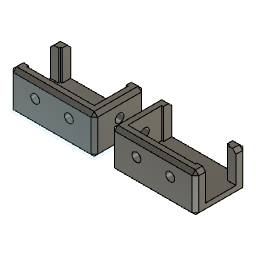
Footv2.5 (Autodesk Fusion 360 design; units mm, degrees)
part number: FootR
part number: FootL
Autodesk Fusion 360 part; units mm, degrees
sketch "Sketch1" plane through (0, 0, 0) normal (0, 0, 1) x (1, 0, 0) in component "FootR"
  line L0 (5, 5) -> (55, 5)
  line L1 (55, 5) -> (55, 35)
  line L2 (55, 35) -> (5, 35)
  line L3 (5, 35) -> (5, 5)
  dimension "d1" = 50
  dimension "d2" = 30
  constraint horizontal L0
  constraint vertical L1
  constraint horizontal L2
  constraint vertical L3
  measures "d1" distance of L0.start L0.end
  measures "d2" distance of L0.start L2.end
extrude "Extrude1" add sketch "Sketch1" along normal blind 23 makes body 1 in component "FootR"
move_body "Move1" bodies 1 to x (1, 0, 0) y (0, 1, 0) z (0, 0, 1) at (3.5577, -2.3008, 1.4706) in component "FootR"
sketch "Sketch1 (2)" plane through (0, 0, 0) normal (0, 0, -1) x (1, 0, 0)
  line L0 (0, 0) -> (0, -30)
  line L1 (0, -30) -> (50, -30)
  line L2 (50, -30) -> (50, 0)
  line L3 (50, 0) -> (0, 0)
sketch "Sketch2" plane through (0, 0, 23) normal (0, 0, 1) x (-1, 0, 0)
  line L0 (0, -30) -> (0, 0)
  line L1 (0, 0) -> (-50, 0)
  line L2 (-50, 0) -> (-50, -30)
  line L3 (-50, -30) -> (0, -30)
  line L4 (-5, -25) -> (-45, -25)
  line L5 (-45, -25) -> (-45, -5)
  line L6 (-45, -5) -> (-5, -5)
  line L7 (-5, -5) -> (-5, -25)
  dimension "d5" = 40
  dimension "d6" = 20
  dimension "d7" = 5
  dimension "d8" = 5
  constraint horizontal L4
  constraint vertical L5
  constraint horizontal L6
  constraint vertical L7
  measures "d5" distance of L4.start L4.end
  measures "d6" distance of L4.start L6.end
  measures "d7" distance of L3 L4
  measures "d8" distance of L2 L5
extrude "Extrude2" cut sketch "Sketch2" against normal blind 18 contours L4 L5 L6 L7 sketch seen with x (1, 0, 0) y (0, 1, 0) z (0, 0, 1) at (8.5577, 2.6992, 1.4706) bodies 1 in component "FootR"
chamfer "Chamfer1" distance 2 angle 45 4 faces at (25.2244, 2.6992, 9.1373) (58.5577, 12.6992, 16.804) (41.8911, 32.6992, 9.1373) (8.5577, 22.6992, 9.1373) on bodies 1 in component "FootR"
sketch "Sketch3" plane through (0, 0, 23) normal (0, 0, 1) x (-1, 0, 0)
  line L0 (-45, -25) -> (-45, -5)
  line L1 (-45, -5) -> (-5, -5)
  line L2 (-5, -5) -> (-5, -25)
  line L3 (-5, -25) -> (-45, -25)
  line L4 (-2, -2) -> (-48, -2)
  line L5 (-48, -2) -> (-48, -28)
  line L6 (-48, -28) -> (-2, -28)
  line L7 (-2, -28) -> (-2, -2)
  line L8 (-6, -25) -> (-44, -25)
  line L9 (-44, -25) -> (-44, -30)
  line L10 (-44, -30) -> (-6, -30)
  line L11 (-6, -30) -> (-6, -25)
  line L12 (-50, -30) -> (-50, 0)
  dimension "d12" = 5
  dimension "d13" = 38
  dimension "d14" = 6
  constraint horizontal L8
  constraint vertical L9
  constraint horizontal L10
  constraint vertical L11
  constraint coincident L3 L8.start
  measures "d12" distance of L8.start L10.end
  measures "d13" distance of L9.end L10.end
  measures "d14" distance of L9 L12
extrude "Extrude3" cut sketch "Sketch3" against normal blind 18 contours L3 L6 L8 L9 L11 | L6 L9 L10 L11 sketch seen with x (1, 0, 0) y (0, 1, 0) z (0, 0, 1) at (8.5577, 2.6992, 1.4706) bodies 1 in component "FootR"
sketch "Sketch4" plane through (0, 0, 23) normal (0, 0, 1) x (-1, 0, 0)
  line L0 (-6, -25) -> (-6, -28)
  line L1 (-6, -28) -> (-2, -28)
  line L2 (-2, -28) -> (-2, -2)
  line L3 (-2, -2) -> (-48, -2)
  line L4 (-48, -2) -> (-48, -28)
  line L5 (-48, -28) -> (-44, -28)
  line L6 (-44, -28) -> (-44, -25)
  line L7 (-44, -25) -> (-45, -25)
  line L8 (-45, -25) -> (-45, -5)
  line L9 (-45, -5) -> (-5, -5)
  line L10 (-5, -5) -> (-5, -25)
  line L11 (-5, -25) -> (-6, -25)
  line L12 (-5, -24) -> (0, -24)
  line L13 (0, -24) -> (0, -6)
  line L14 (0, -6) -> (-5, -6)
  line L15 (-5, -6) -> (-5, -24)
  line L16 (-50, 0) -> (0, 0)
  dimension "d17" = 5
  dimension "d18" = 6
  dimension "d19" = 18
  constraint horizontal L12
  constraint vertical L13
  constraint horizontal L14
  constraint vertical L15
  constraint coincident L10 L12.start
  measures "d17" distance of L13 L15
  measures "d18" distance of L14 L16
  measures "d19" distance of L12 L14
extrude "Extrude4" cut sketch "Sketch4" against normal blind 18 contours L2 L10 L12 L14 L15 | L2 L12 L13 L14 sketch seen with x (1, 0, 0) y (0, 1, 0) z (0, 0, 1) at (8.5577, 2.6992, 1.4706) bodies 1 in component "FootR"
sketch "Sketch5" plane through (45, 0, 0) normal (-1, 0, 0) x (0, -1, 0)
  line L0 (-5, 23) -> (-25, 23)
  line L1 (-25, 23) -> (-25, 5)
  line L2 (-25, 5) -> (-5, 5)
  line L3 (-5, 5) -> (-5, 23)
  circle A0 centre (-15, 14) radius 2.6
  dimension "d22" = 5.2
  dimension "d23" = 10
  dimension "d24" = 9
  measures "d22" diameter of A0
  measures "d23" distance of L1 A0.centre
  measures "d24" distance of L2 A0.centre
extrude "Extrude5" cut sketch "Sketch5" against normal blind 5 contours A0 sketch seen with x (1, 0, 0) y (0, 1, 0) z (0, 0, 1) at (8.5577, 2.6992, 1.4706) bodies 1 in component "FootR"
sketch "Sketch6" plane through (0, 5, 0) normal (0, 1, 0) x (-1, 0, 0)
  line L0 (-5, 23) -> (-45, 23)
  line L1 (-45, 23) -> (-45, 5)
  line L2 (-45, 5) -> (-5, 5)
  line L3 (-5, 5) -> (-5, 23)
  circle A0 centre (-35, 14) radius 2.6
  circle A1 centre (-15, 14) radius 2.6
  dimension "d27" = 5.2
  dimension "d28" = 10
  dimension "d29" = 9
  dimension "d30" = 5.2
  dimension "d31" = 10
  dimension "d32" = 9
  measures "d27" diameter of A0
  measures "d28" distance of L1 A0.centre
  measures "d29" distance of L2 A0.centre
  measures "d30" diameter of A1
  measures "d31" distance of L3 A1.centre
  measures "d32" distance of L2 A1.centre
extrude "Extrude6" cut sketch "Sketch6" against normal blind 5 contours A0 | A1 sketch seen with x (1, 0, 0) y (0, 1, 0) z (0, 0, 1) at (8.5577, 2.6992, 1.4706) bodies 1 in component "FootR"
mirror "MirrorComponent1" about plane through (0, 0, 0) normal (0, 0, 1) of bodies 1 makes body 2 in component "FootL"
sketch "Sketch7" plane through (0, 0, 0) normal (0, -1, 0) x (1, 0, 0)
  circle A0 centre (35, 14) radius 2.6
  circle A1 centre (15, 14) radius 2.6
  line L0 (2, 2) -> (48, 2)
  line L1 (48, 2) -> (48, 21)
  line L2 (48, 21) -> (2, 21)
  line L3 (2, 21) -> (2, 2)
component "FootR" placed x (1, 0, 0) y (0, 1, 0) z (0, 0, 1) at (-8.5577, -2.6992, -1.4706)
component "FootL" placed x (-1, 0, 0) y (0, 1, 0) z (0, 0, -1) at (108.5577, -2.6992, -1.4706)
